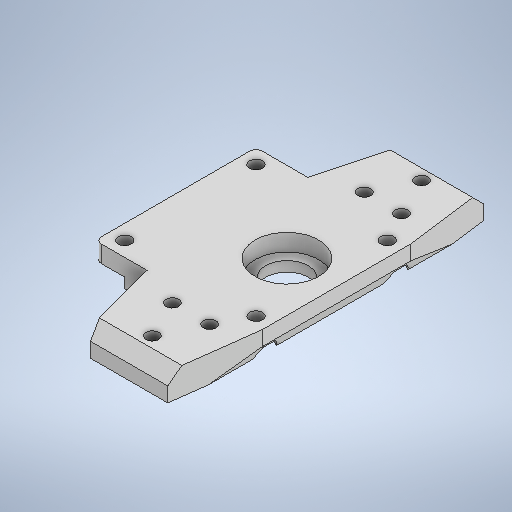
# Autodesk Inventor part: Honigschleuder
Saved by Autodesk Inventor 2025 (Build 290162010, 162A)
## iProperties
Created: 2025-11-15
Part Number: Honigschleuder
Material: Generisch
Document SubType Name: Modeling
Designer: max-h
Density: 1 g/cm^3
Appearance: Vorgabe
Author: max-h
Autodesk Inventor part; units mm, degrees
ref_plane "YZ Plane" through (0, 0, 0) normal (1, 0, 0) x (0, 1, 0)
ref_plane "XZ Plane" through (0, 0, 0) normal (0, 1, 0) x (-1, 0, 0)
ref_plane "XY Plane" through (0, 0, 0) normal (0, 0, 1) x (1, 0, 0)
sketch "Skizze1" plane through (0, 0, 0) normal (0, 1, 0) x (-1, 0, 0)
  line L0 (48, 52) -> (-48, 52)
  line L1 (-52, 48) -> (-52, -48)
  line L2 (-48, -52) -> (48, -52)
  line L3 (52, -48) -> (52, 48)
  arc A0 (52, 48) -> (48, 52) centre (48, 48) ccw
  arc A1 (48, -52) -> (52, -48) centre (48, -48) ccw
  arc A2 (-52, -48) -> (-48, -52) centre (-48, -48) ccw
  arc A3 (-48, 52) -> (-52, 48) centre (-48, 48) ccw
  line L4 (52, 48) -> (48, 48) construction
  line L5 (48, 48) -> (48, 52) construction
  line L6 (52, -48) -> (48, -48) construction
  line L7 (48, -48) -> (48, -52) construction
  line L8 (-48, -52) -> (-48, -48) construction
  line L9 (-48, -48) -> (-52, -48) construction
  line L10 (-48, 52) -> (-48, 48) construction
  line L11 (-52, 48) -> (-48, 48) construction
  line L12 (84, 0) -> (-84, 0) construction
  line L13 (0, -170.5701) -> (0, 153.9024) construction
  circle A4 centre (0, 0) radius 60 construction
  circle A5 centre (42.4264, -42.4264) radius 4.25
  circle A6 centre (-42.4264, -42.4264) radius 4.25
  circle A7 centre (-42.4264, 42.4264) radius 4.25
  circle A8 centre (42.4264, 42.4264) radius 4.25
  line L14 (42.4264, 42.4264) -> (-42.4264, 42.4264) construction
  line L15 (-42.4264, 42.4264) -> (-42.4264, -42.4264) construction
  line L16 (-42.4264, -42.4264) -> (42.4264, -42.4264) construction
  line L17 (42.4264, -42.4264) -> (42.4264, 42.4264) construction
  line L18 (42.4264, -42.4264) -> (42.4264, -52) construction
  line L19 (42.4264, -42.4264) -> (52, -42.4264) construction
  line L20 (5, 107.5492) -> (-45, 107.5492) construction
  line L21 (-45, 107.5492) -> (-45, -124.2169) construction
  line L22 (-45, -124.2169) -> (5, -124.2169) construction
  line L23 (5, -124.2169) -> (5, 107.5492) construction
  circle A9 centre (-20, 0) radius 13.75
  line L24 (-20, 18.0436) -> (-20, -25.5729)
  line L25 (18.3975, 52) -> (5, 102)
  line L26 (5, 102) -> (-45, 102)
  line L27 (-45, 102) -> (-52, 48)
  line L28 (18.3975, -52) -> (5, -102)
  line L29 (-45, -102) -> (-52, -48)
  line L30 (5, -102) -> (-45, -102)
  circle A10 centre (-20, 87) radius 4.1
  circle A11 centre (-20, 69) radius 4.1 construction
  circle A12 centre (-20, -69) radius 4.1 construction
  circle A13 centre (-20, -87) radius 4.1
  circle A14 centre (-32, 62) radius 4.1
  circle A15 centre (-8, 62) radius 4.1
  circle A16 centre (-8, -62) radius 4.1
  circle A17 centre (-32, -62) radius 4.1
  point P0 (0, 52)
  point P1 (0, -52)
  dimension "d1" = 104
  dimension "d2" = 120
  dimension "d3" = 8.5
  dimension "d4" = 4
  dimension "d5" = 50
  dimension "d6" = 20
  dimension "d7" = 27.5
  dimension "d9" = 50
  dimension "d10" = 50
  dimension "d13" = 75
  dimension "d14" = 75
  dimension "d17" = 8.2
  dimension "d18" = 18
  dimension "d19" = 15
  dimension "d20" = 18
  dimension "d21" = 15
  dimension "d22" = 12
  dimension "d23" = 7
  dimension "d24" = 12
  dimension "d25" = 7
  dimension "d26" = 7
  dimension "d27" = 7
  dimension "d28" = 12
  dimension "d29" = 12
  constraints: 58 end point, 18 centre point, 14 point on line, 13 equal radius, 12 perpendicular, 12 point on circle, 6 horizontal, 6 parallel, 5 coincident, 3 vertical, 2 midpoint, 3 other
  measures "d1" distance between parallel lines of L0 L2
  measures "d2" diameter of A4
  measures "d3" diameter of A8
  measures "d4" distance of L3.start L6.end
  measures "d5" distance of L21.end L22.end
  measures "d6" distance from line of L13 A9.centre
  measures "d7" diameter of A9
  measures "d9" distance between parallel lines of L0 L26
  measures "d10" distance between parallel lines of L30 L2
  measures "d13" angle of L0 L25
  measures "d14" angle of L2 L28
  measures "d17" diameter of A10
  measures "d18" distance of A11.centre A10.centre
  measures "d19" distance from line of L26 A10.centre
  measures "d20" distance of A13.centre A12.centre
  measures "d21" distance from line of L30 A13.centre
  measures "d22" horizontal distance of A11.centre A14.centre
  measures "d23" vertical distance of A11.centre A14.centre
  measures "d24" horizontal distance of A11.centre A15.centre
  measures "d25" vertical distance of A15.centre A11.centre
  measures "d26" vertical distance of A12.centre A17.centre
  measures "d27" vertical distance of A12.centre A16.centre
  measures "d28" horizontal distance of A12.centre A16.centre
  measures "d29" horizontal distance of A12.centre A17.centre
extrude "Extrusion1" add sketch "Skizze1" along normal blind 17.5 contours A0 L3 A1 L2 A2 L29 L1 L27 A3 L0 | L0 A3 L27 L26 L25 | L28 L30 L29 A2 L2
sketch "Skizze2" plane through (0, 17.5, 0) normal (0, 1, 0) x (1, 0, 0)
  circle A0 centre (20, 0) radius 13.75 projected
  circle A1 centre (20, 0) radius 20.5
  point P0 (0, 0)
  dimension "d30" = 41
  constraints: 1 centre point, 1 coincident
  measures "d30" diameter of A1
extrude "Extrusion2" cut sketch "Skizze2" against normal blind 11
sketch "Skizze3" plane through (0, 0, 0) normal (0, -1, 0) x (1, 0, 0)
  circle A0 centre (-42.4264, -42.4264) radius 4.25 projected
  circle A1 centre (42.4264, -42.4264) radius 4.25 projected
  circle A2 centre (42.4264, 42.4264) radius 4.25 projected
  circle A3 centre (-42.4264, 42.4264) radius 4.25 projected
  arc A4 (-42.4264, 32.9264) -> (-32.9264, 42.4264) centre (-42.4264, 42.4264) ccw
  circle A5 centre (42.4264, 42.4264) radius 9.5
  circle A6 centre (42.4264, -42.4264) radius 9.5
  circle A7 centre (-42.4264, -42.4264) radius 4.25 projected
  arc A8 (-32.9264, -42.4264) -> (-42.4264, -32.9264) centre (-42.4264, -42.4264) ccw
  line L0 (-42.4264, -32.9264) -> (-52, -32.9264)
  line L1 (-52, -48) -> (-52, 48) projected
  line L2 (-42.4264, -32.9264) -> (-42.4264, -42.4264) construction
  line L3 (-42.4264, -42.4264) -> (-32.9264, -42.4264) construction
  line L4 (-32.9264, -42.4264) -> (-32.9264, -52)
  line L5 (-18.3975, -52) -> (-48, -52) projected
  line L6 (-32.9264, 42.4264) -> (-32.9264, 52)
  line L7 (-42.4264, 32.9264) -> (-52, 32.9264)
  line L8 (-48, 52) -> (-18.3975, 52) projected
  arc A9 (-52, -48) -> (-48, -52) centre (-48, -48) ccw projected
  arc A10 (-48, 52) -> (-52, 48) centre (-48, 48) ccw projected
  point P0 (0, 0)
  dimension "d36" = 19
  constraints: 12 end point, 5 point on circle, 4 centre point, 4 coincident, 4 point on line, 3 equal radius, 3 horizontal, 2 tangent, 2 vertical, 1 parallel
  measures "d36" diameter of A8
extrude "Extrusion3" cut sketch "Skizze3" against normal blind 6.5
chamfer "Fasen2" distance 8 distance2 4 1 edges at (52, 0, 0) measured on face at (52, 0.5, 0)
chamfer "Fasen3" distance 8 angle 45 2 edges at (20, 17.5, 102) (20, 17.5, -102)
